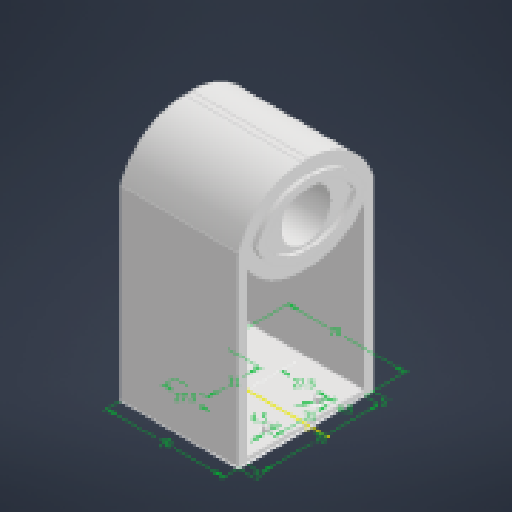
# Autodesk Inventor part: Part13
Saved by Autodesk Inventor 2027 (Build 310192060, 192F)
## iProperties
Created: 2026-08-17
Part Number: Part13
Material: Generic
Document SubType Name: Modeling
Designer: trtrn
Density: 1 g/cm^3
Appearance: Default
Author: trtrn
Autodesk Inventor part; units mm, degrees
ref_plane "YZ Plane" through (0, 0, 0) normal (1, 0, 0) x (0, 1, 0)
ref_plane "XZ Plane" through (0, 0, 0) normal (0, 1, 0) x (-1, 0, 0)
ref_plane "XY Plane" through (0, 0, 0) normal (0, 0, 1) x (1, 0, 0)
sketch "Sketch1" plane through (0, 0, 0) normal (0, 1, 0) x (-1, 0, 0)
  line L0 (35, 35) -> (-35, 35)
  line L1 (-35, 35) -> (-35, -35)
  line L2 (-35, -35) -> (35, -35)
  line L3 (35, -35) -> (35, 35)
  line L4 (35, 35) -> (-35, -35) construction
  line L5 (-35, 35) -> (35, -35) construction
  line L6 (35, 35) -> (-35, 35)
  line L7 (-35, 35) -> (-35, 40)
  line L8 (-35, 40) -> (35, 40)
  line L9 (35, 40) -> (35, 35)
  line L10 (35, -35) -> (-35, -35)
  line L11 (-35, -35) -> (-35, -40)
  line L12 (-35, -40) -> (35, -40)
  line L13 (35, -40) -> (35, -35)
  point P0 (0, 0)
  dimension "d0" = 70
  dimension "d1" = 70
  dimension "d2" = 70
  dimension "d3" = 5
  dimension "d4" = 5
  constraints: 28 end point, 6 parallel, 3 horizontal, 3 perpendicular, 2 midpoint, 1 point on line
  measures "d0" distance of L1.end L0.end
  measures "d1" distance between parallel lines of L1 L3
  measures "d2" distance of L7.end L8.end
  measures "d3" distance of L6.end L7.end
  measures "d4" distance of L11.end L10.end
extrude "Extrusion1" add sketch "Sketch1" along normal blind 3 contours L3 L2 L1 L0
extrude "Extrusion2" add sketch "Sketch1" along normal blind 110.75 contours L0 L7 L8 L9 | L13 L12 L11 L2
sketch "Sketch2" plane through (0, 3, 0) normal (0, 1, 0) x (1, 0, 0)
  line L0 (-49, 0) -> (49, 0) projected
  line L1 (0, -23.8249) -> (0, 29.3296) construction
  circle A0 centre (27.5, -15.5) radius 2.25
  circle A1 centre (27.5, 15.5) radius 2.25
  point P0 (0, 0)
  point P1 (-27.5, -15.5)
  point P2 (-27.5, 15.5)
  dimension "d9" = 31
  dimension "d11" = 27.5
  dimension "d19" = 27.5
  dimension "d20" = 31
  dimension "d21" = 4.5
  dimension "d22" = 4.5
  constraints: 2 centre point, 2 coincident, 2 end point, 2 symmetric about line, 2 vertical alignment, 1 point on line, 1 vertical
  measures "d9" distance of point (-27.5, -15.5) point (-27.5, 15.5)
  measures "d11" distance from line of L1 point (-27.5, -15.5)
  measures "d19" distance from line of L1 point (27.5, 15.5)
  measures "d20" distance of point (27.5, -15.5) point (27.5, 15.5)
  measures "d21" diameter of A0
  measures "d22" diameter of A1
hole "Hole1" at (-27.5, 3, -15.5) at (-27.5, 3, 15.5) direction (0, -1, 0) diameter 5 end through all
extrude "Extrusion3" add sketch "Sketch2" along normal blind 3
sketch "Sketch3" plane through (35, 0, 40) normal (1, 0, 0) x (0, 0, -1)
  circle A0 centre (40, 110.75) radius 15
  line L0 (75, 110.75) -> (80, 110.75) projected
  line L1 (0, 110.75) -> (5, 110.75) projected
  line L2 (0, 0) -> (80, 0) projected
  arc A1 (80, 110.75) -> (0, 110.75) centre (40, 80.75) ccw
  arc A2 (0, 110.75) -> (80, 110.75) centre (40, 140.75) ccw
  line L3 (25, 110.75) -> (55, 110.75) construction
  point P0 (40, 0)
  point P1 (77.5, 110.75)
  point P2 (40, 0)
  point P3 (40, 110.75)
  point P4 (40, 130.75)
  dimension "d25" = 30
  dimension "d26" = 20
  constraints: 7 point on circle, 4 end point, 4 midpoint, 3 centre point, 1 horizontal, 1 horizontal alignment, 1 symmetric about line, 1 vertical alignment
  measures "d25" diameter of A0
  measures "d26" distance of point (40, 110.75) point (40, 130.75)
extrude "Extrusion4" add sketch "Sketch3" against normal up to surface (70 mm away)
sketch "Sketch4" plane through (35, 0, 40) normal (1, 0, 0) x (0, 0, -1)
  point P0 (40, 0)
sketch "Sketch5" plane through (35, 0, 40) normal (1, 0, 0) x (0, 0, -1)
  arc A0 (42, 94.75) -> (67.2982, 110.75) centre (42, 122.75) ccw projected
  arc A1 (67.2982, 110.75) -> (42, 126.75) centre (42, 98.75) ccw projected
  arc A2 (38, 126.75) -> (12.7018, 110.75) centre (38, 98.75) ccw projected
  arc A3 (12.7018, 110.75) -> (38, 94.75) centre (38, 122.75) ccw projected
  line L0 (42, 126.75) -> (40, 126.75) projected
  line L1 (40, 126.75) -> (38, 126.75) projected
  line L2 (40, 94.75) -> (42, 94.75) projected
  line L3 (38, 94.75) -> (40, 94.75) projected
  arc A4 (80, 110.75) -> (42, 138.5997) centre (42, 98.75) ccw
  arc A5 (42, 82.9003) -> (80, 110.75) centre (42, 122.75) ccw
  line L4 (42, 82.9003) -> (40, 82.9003)
  line L5 (40, 82.9003) -> (38, 82.9003)
  arc A6 (0, 110.75) -> (38, 82.9003) centre (38, 122.75) ccw
  arc A7 (38, 138.5997) -> (0, 110.75) centre (38, 98.75) ccw
  line L6 (38, 138.5997) -> (40, 138.5997)
  line L7 (40, 138.5997) -> (42, 138.5997)
  arc A8 (67.2982, 110.75) -> (42, 126.75) centre (42, 98.75) ccw
  arc A9 (42, 94.75) -> (67.2982, 110.75) centre (42, 122.75) ccw
  line L8 (42, 94.75) -> (40, 94.75)
  line L9 (40, 94.75) -> (38, 94.75)
  arc A10 (12.7018, 110.75) -> (38, 94.75) centre (38, 122.75) ccw
  arc A11 (38, 126.75) -> (12.7018, 110.75) centre (38, 98.75) ccw
  line L10 (38, 126.75) -> (40, 126.75)
  line L11 (40, 126.75) -> (42, 126.75)
  point P0 (40, 0)
  constraints: 16 end point, 16 point on circle, 8 centre point, 1 coincident, 14 other
extrude "Extrusion5" add sketch "Sketch5" against normal up to surface (70 mm away)
sketch "Sketch6" plane through (35, 0, 40) normal (1, 0, 0) x (0, 0, -1)
  arc A0 (42, 94.75) -> (67.2982, 110.75) centre (42, 122.75) ccw projected
  arc A1 (67.2982, 110.75) -> (42, 126.75) centre (42, 98.75) ccw projected
  arc A2 (38, 126.75) -> (12.7018, 110.75) centre (38, 98.75) ccw projected
  arc A3 (12.7018, 110.75) -> (38, 94.75) centre (38, 122.75) ccw projected
  line L0 (38, 94.75) -> (42, 94.75) projected
  line L1 (42, 126.75) -> (38, 126.75) projected
  arc A4 (67.2982, 110.75) -> (42, 126.75) centre (42, 98.75) ccw
  arc A5 (42, 94.75) -> (67.2982, 110.75) centre (42, 122.75) ccw
  line L2 (42, 94.75) -> (38, 94.75)
  arc A6 (12.7018, 110.75) -> (38, 94.75) centre (38, 122.75) ccw
  arc A7 (38, 126.75) -> (12.7018, 110.75) centre (38, 98.75) ccw
  line L3 (38, 126.75) -> (42, 126.75)
  arc A8 (72.2982, 110.75) -> (42, 131.3381) centre (42, 98.75) ccw
  arc A9 (42, 90.1619) -> (72.2982, 110.75) centre (42, 122.75) ccw
  line L4 (42, 90.1619) -> (38, 90.1619)
  arc A10 (7.7018, 110.75) -> (38, 90.1619) centre (38, 122.75) ccw
  arc A11 (38, 131.3381) -> (7.7018, 110.75) centre (38, 98.75) ccw
  line L5 (38, 131.3381) -> (42, 131.3381)
  point P0 (40, 0)
  dimension "d31" = 5
  constraints: 16 point on circle, 8 centre point, 8 end point, 10 other
  measures "d31" distance of A0.end A8.start
extrude "Extrusion6" add sketch "Sketch6" along normal blind 3
body "Solid1"
